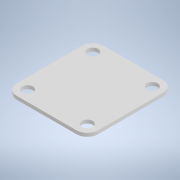
# Autodesk Inventor part: micro lipo footprint
Saved by Autodesk Inventor 2020 (Build 240168000, 168)
## iProperties
Created: 2020-08-31
Part Number: micro lipo footprint
Material: Generic
Document SubType Name: Modeling
Designer: mulve
Density: 1 g/cm^3
Appearance: Default
Author: mulve
Autodesk Inventor part; units mm, degrees
ref_plane "YZ Plane" through (0, 0, 0) normal (1, 0, 0) x (0, 1, 0)
ref_plane "XZ Plane" through (0, 0, 0) normal (0, 1, 0) x (-1, 0, 0)
ref_plane "XY Plane" through (0, 0, 0) normal (0, 0, 1) x (1, 0, 0)
sketch "Sketch1" plane through (0, 0, 0) normal (0, 1, 0) x (-1, 0, 0)
  line L0 (0, 0) -> (19.05, 0)
  line L1 (19.05, 0) -> (19.05, -20.32)
  line L2 (19.05, -20.32) -> (0, -20.32)
  line L3 (0, -20.32) -> (0, 0)
  circle A0 centre (16.51, -2.54) radius 1.2639
  circle A1 centre (16.51, -17.78) radius 1.27
  circle A2 centre (2.54, -17.78) radius 1.27
  circle A3 centre (2.54, -2.54) radius 1.27
  dimension "d0" = 20.32
  dimension "d1" = 19.05
  dimension "d2" = 15.24
  dimension "d3" = 2.54
  dimension "d4" = 15.24
  dimension "d5" = 13.97
  dimension "d6" = 2.54
  dimension "d7" = 13.97
  dimension "d8" = 2.54
  dimension "d9" = 2.54
  dimension "d10" = 2.54
  dimension "d11" = 2.54
  dimension "d12" = 2.54
  dimension "d13" = 2.54
  constraints: 8 end point, 4 centre point, 4 coincident, 2 parallel, 1 horizontal, 1 perpendicular
  measures "d0" distance of L0.end L1.end
  measures "d1" distance of L1.end L2.end
  measures "d2" distance of point (16.51, -17.78) point (16.51, -2.54)
  measures "d3" distance from line of L0 point (16.51, -2.54)
  measures "d4" distance of point (2.54, -17.78) point (2.54, -2.54)
  measures "d5" distance of point (16.51, -17.78) point (2.54, -17.78)
  measures "d6" distance from line of L1 point (16.51, -17.78)
  measures "d7" distance of point (2.54, -2.54) point (16.51, -2.54)
  measures "d8" distance from line of L3 point (2.54, -17.78)
  measures "d9" distance from line of L3 point (2.54, -2.54)
  measures "d10" distance from line of L1 point (16.51, -2.54)
  measures "d11" diameter of A1
  measures "d12" diameter of A2
  measures "d13" diameter of A3
extrude "Extrusion1" add sketch "Sketch1" along normal blind 0.8
fillet "Fillet1" radius 2.54 4 edges at (0, 0.4, 0) (0, 0.4, -20.32) (-19.05, 0.4, -20.32) (-19.05, 0.4, 0)
equation "\"d7\" = d5"
equation "\"d9\" = d8"
body "Solid1"
